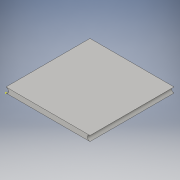
# Autodesk Inventor part: peltier_module
Saved by Autodesk Inventor 2016 (Build 200138000, 138)
## iProperties
Created: 2016-02-26
Part Number: peltier_module
Material: Generic
Document SubType Name: Modeling
Designer: USKHNGO
Density: 1 g/cm^3
Appearance: Default
Author: USKHNGO
Autodesk Inventor part; units mm, degrees
ref_plane "YZ Plane" through (0, 0, 0) normal (1, 0, 0) x (0, 1, 0)
ref_plane "XZ Plane" through (0, 0, 0) normal (0, 1, 0) x (-1, 0, 0)
ref_plane "XY Plane" through (0, 0, 0) normal (0, 0, 1) x (1, 0, 0)
sketch "Sketch1" plane through (0, 0, 0) normal (0, 1, 0) x (-1, 0, 0)
  point P0 (0, 0)
sketch "Sketch2" plane through (0, 0, 0) normal (0, 0, 1) x (1, 0, 0)
  line L0 (0, 0) -> (62, 0)
  line L1 (62, 3.9) -> (0, 3.9)
  arc A0 (0, 0) -> (0, 3.9) centre (0, 1.95) ccw
  arc A1 (62, 3.9) -> (62, 0) centre (62, 1.95) ccw
  dimension "d0" = 62
  dimension "d1" = 3.9
  constraints: 4 end point, 4 point on circle, 4 tangent, 2 centre point, 1 horizontal, 1 parallel
  measures "d0" distance of L1.end L1.start
  measures "d1" distance of L1.start L0.end
extrude "Extrusion1" add sketch "Sketch2" against normal blind 62
body "Solid1"
